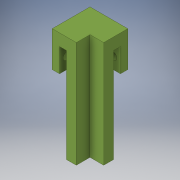
# Autodesk Inventor part: TelescopeGroot 8
Saved by Autodesk Inventor 2018.3 (Build 223284000, 284)
## iProperties
Created: 2020-01-26
Part Number: TelescopeGroot 8
Material: Generic
Document SubType Name: Modeling
Designer: 21roosmich
Density: 1 g/cm^3
Appearance: Olive Green
Mass: 6.75159 g
Surface Area: 48.2134 cm^2
Volume: 6.75159 cm^3
Author: 21roosmich
Autodesk Inventor part; units mm, degrees
ref_plane "YZ Plane" through (0, 0, 0) normal (1, 0, 0) x (0, 1, 0)
ref_plane "XZ Plane" through (0, 0, 0) normal (0, 1, 0) x (-1, 0, 0)
ref_plane "XY Plane" through (0, 0, 0) normal (0, 0, 1) x (1, 0, 0)
sketch "Sketch1" plane through (0, 0, 0) normal (0, 1, 0) x (-1, 0, 0)
  line L0 (0, 0) -> (-2.54, 0)
  line L1 (-2.54, 0) -> (-2.54, -12.7)
  line L2 (-2.54, -12.7) -> (0, -12.7)
  line L3 (0, -12.7) -> (0, 0)
  line L4 (0, -12.7) -> (-12.7, -12.7)
  line L5 (-12.7, -12.7) -> (-12.7, -10.16)
  line L6 (-12.7, -10.16) -> (0, -10.16)
  line L7 (0, -10.16) -> (0, -12.7)
  dimension "d0" = 12.7
  dimension "d1" = 12.7
  dimension "d2" = 2.54
  dimension "d3" = 2.54
  constraints: 16 end point, 4 parallel, 2 horizontal, 2 perpendicular
  measures "d0" distance of L2.end L4.end
  measures "d1" distance of L2.end L0.start
  measures "d2" distance of L4.end L5.end
  measures "d3" distance of L0.start L0.end
extrude "Extrusion1" add sketch "Sketch1" along normal blind 50.8
sketch "Sketch2" plane through (0, 50.8, 0) normal (0, 1, 0) x (1, 0, 0)
  line L0 (2.54, 0) -> (-7.62, 0)
  line L1 (-7.62, 0) -> (-7.62, 20.32)
  line L2 (-7.62, 20.32) -> (2.54, 20.32)
  line L3 (2.54, 20.32) -> (2.54, 0)
  line L4 (12.7, 10.16) -> (12.7, 12.7) projected
  line L5 (12.7, 10.16) -> (-7.62, 10.16)
  line L6 (-7.62, 10.16) -> (-7.62, 20.32)
  line L7 (-7.62, 20.32) -> (12.7, 20.32)
  line L8 (12.7, 20.32) -> (12.7, 10.16)
  line L9 (2.54, 0) -> (2.54, 10.16) projected
  point P0 (0, 0)
  dimension "d6" = 10.16
  dimension "d7" = 0
  dimension "d8" = 10.16
  dimension "d9" = 20.32
  constraints: 16 end point, 4 parallel, 2 horizontal, 2 perpendicular
  measures "d6" distance of L0.start L0.end
  measures "d7" distance between parallel lines of L9 L3
  measures "d8" distance of L7.end L4.start
  measures "d9" distance between parallel lines of L2 L0
extrude "Extrusion2" add sketch "Sketch2" along normal blind 6.35
sketch "Sketch3" plane through (0, 50.8, 0) normal (0, -1, 0) x (1, 0, 0)
  line L0 (-7.62, -20.32) -> (12.7, -20.32) projected
  line L1 (12.7, -20.32) -> (-7.62, -20.32)
  line L2 (-7.62, -20.32) -> (-7.62, -16.383)
  line L3 (-7.62, -16.383) -> (12.7, -16.383)
  line L4 (12.7, -16.383) -> (12.7, -20.32)
  line L5 (-7.62, 0) -> (-3.683, 0)
  line L6 (-3.683, 0) -> (-3.683, -20.32)
  line L7 (-3.683, -20.32) -> (-7.62, -20.32)
  line L8 (-7.62, -20.32) -> (-7.62, 0)
  line L9 (0, -12.7) -> (0, 0) projected
  line L10 (12.7, -12.7) -> (0, -12.7) projected
  dimension "d12" = 3.683
  dimension "d13" = 3.683
  constraints: 16 end point, 4 parallel, 2 horizontal, 2 perpendicular, 2 point on line
  measures "d12" distance between parallel lines of L6 L9
  measures "d13" distance between parallel lines of L10 L3
extrude "Extrusion3" add sketch "Sketch3" along normal blind 12.7
sketch "Sketch4" plane through (-7.62, 57.15, -20.32) normal (-1, 0, 0) x (0, 0, 1)
  line L0 (20.32, 0) -> (20.32, -19.05) projected
  line L1 (0, 0) -> (20.32, 0) projected
  point P0 (20.32, -57.15)
  point P1 (16.51, -12.7)
  point P2 (20.32, -6.35)
  dimension "d16" = 3.81
  dimension "d27" = 6.35
  measures "d16" distance from line of L0 point (16.51, -12.7)
  measures "d27" vertical distance of point (16.51, -12.7) point (20.32, -6.35)
hole "Hole1" at (-7.62, 44.45, -3.81) direction (1, 0, 0) diameter 3.81 depth 4.318 tip angle 118
sketch "Sketch5" plane through (12.7, 57.15, -20.32) normal (0, 0, -1) x (-1, 0, 0)
  line L0 (16.383, -6.35) -> (0, -6.35) projected
  line L1 (0, 0) -> (0, -19.05) projected
  point P0 (12.7, -57.15)
  point P1 (3.81, -12.7)
  dimension "d28" = 6.35
  dimension "d29" = 3.81
  measures "d28" distance from line of L0 point (3.81, -12.7)
  measures "d29" distance from line of L1 point (3.81, -12.7)
hole "Hole2" at (8.89, 44.45, -20.32) direction (0, 0, 1) diameter 3.81 depth 4.445 tip angle 118
sketch "Sketch6" plane through (0, 0, 0) normal (0, 1, 0) x (-1, 0, 0)
  line L0 (-2.54, 0) -> (-2.54, -10.16) projected
  line L1 (-2.54, 0) -> (-5.334, 0)
  line L2 (-5.334, 0) -> (-5.334, -10.16)
  line L3 (-5.334, -10.16) -> (-2.54, -10.16)
  line L4 (-2.54, -10.16) -> (-2.54, 0)
  line L5 (-2.54, -10.16) -> (-12.7, -10.16) projected
  line L6 (-12.7, -10.16) -> (-2.54, -10.16)
  line L7 (-2.54, -10.16) -> (-2.54, -7.366)
  line L8 (-2.54, -7.366) -> (-12.7, -7.366)
  line L9 (-12.7, -7.366) -> (-12.7, -10.16)
  point P0 (0, 0)
  dimension "d37" = 2.794
  dimension "d38" = 2.794
  constraints: 16 end point, 4 parallel, 2 horizontal, 2 perpendicular, 1 point on line
  measures "d37" distance of L0.start L1.end
  measures "d38" distance of L8.end L5.end
extrude "Extrusion4" add sketch "Sketch6" along normal blind 57.15
equation "\"d38\" = d37"
body "Solid1"
